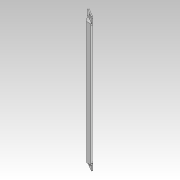
# Autodesk Inventor part: LedBracket
Saved by Autodesk Inventor 2020 (Build 240168000, 168)
## iProperties
Created: 2021-09-12
Part Number: LedBracket
Material: Generic
Document SubType Name: Modeling
Designer: DDeGo
Density: 1 g/cm^3
Appearance: Default
Author: DDeGo
Autodesk Inventor part; units mm, degrees
ref_plane "YZ Plane" through (0, 0, 0) normal (1, 0, 0) x (0, 1, 0)
ref_plane "XZ Plane" through (0, 0, 0) normal (0, 1, 0) x (-1, 0, 0)
ref_plane "XY Plane" through (0, 0, 0) normal (0, 0, 1) x (1, 0, 0)
sketch "Sketch1" plane through (0, 0, 0) normal (0, 0, 1) x (1, 0, 0)
  line L0 (-4, -105) -> (4, -105)
  line L1 (4, -105) -> (4, 105)
  line L2 (4, 105) -> (-4, 105)
  line L3 (-4, 105) -> (-4, -105)
  line L4 (-4, -105) -> (4, 105) construction
  line L5 (4, -105) -> (-4, 105) construction
  point P0 (0, 0)
  dimension "d0" = 8
  dimension "d1" = 210
  constraints: 12 end point, 2 midpoint, 2 parallel, 1 horizontal, 1 perpendicular
  measures "d0" distance of L1.end L2.end
  measures "d1" distance between parallel lines of L0 L2
extrude "Extrusion1" add sketch "Sketch1" along normal blind 2
sketch "Sketch2" plane through (-4, 105, 0) normal (0, 1, 0) x (1, 0, 0)
  line L0 (8, 0) -> (8, -2) projected
  line L1 (8, -2) -> (9.25, 0.1651)
  line L2 (9.25, 0.1651) -> (-8.0705, 10.1651)
  line L3 (8, -2) -> (0, -2) projected
  line L4 (0, 0) -> (0, -2) projected
  line L5 (8, -2) -> (0, -2)
  line L6 (0, -2) -> (-8.8205, 8.866)
  line L7 (-8.8205, 8.866) -> (-8.0705, 10.1651)
  point P0 (4, 0)
  dimension "d4" = 30
  dimension "d5" = 2.5
  dimension "d6" = 20
  dimension "d9" = 1.5
  constraints: 10 end point, 3 perpendicular
  measures "d4" angle of L2 L3
  measures "d5" distance from line of L0.end L2
  measures "d6" distance of L1.end L2.end
  measures "d9" distance of L6.end L2.end
extrude "Extrusion2" add sketch "Sketch2" along normal blind 2
sketch "Sketch3" plane through (-4, 107, 0) normal (0, 1, 0) x (1, 0, 0)
  line L0 (9.25, 0.1651) -> (-8.0705, 10.1651) projected
  line L1 (-8.8205, 8.866) -> (0, -2) projected
  line L2 (-8.0705, 10.1651) -> (-8.8205, 8.866)
  line L3 (-8.8205, 8.866) -> (8.5, -1.134)
  line L4 (8.5, -1.134) -> (9.25, 0.1651)
  line L5 (9.25, 0.1651) -> (-8.0705, 10.1651)
  line L6 (8, -2) -> (9.25, 0.1651) projected
  point P0 (4, 0)
  point P1 (9.25, 0.1651)
  constraints: 8 end point, 2 parallel, 1 perpendicular, 1 point on line
extrude "Extrusion3" add sketch "Sketch3" along normal blind 10
sketch "Sketch4" plane through (4.5, 107, 1.134) normal (-0.5, 0, 0.8660254) x (0.8660254, 0, 0.5)
  line L0 (-20, -2) -> (-20, 10) construction
  line L1 (-6.9282, 0) -> (0, 0) projected
  line L2 (-20, 10) -> (0, 0) construction
  circle A0 centre (-10, 5) radius 2.75
  point P0 (-4.4641, -107)
  dimension "d12" = 5.5
  constraints: 2 end point, 1 centre point, 1 midpoint
  measures "d12" diameter of A0
extrude "Extrusion4" cut sketch "Sketch4" against normal blind 10
fillet "Fillet1" radius 2 2 edges at (-12.4455, 117, -9.5155) (4.875, 117, 0.4845)
fillet "Fillet2" radius 5 1 edges at (0, 105, 0)
mirror "Mirror1" about plane through (0, 0, 0) normal (0, 1, 0) of "Extrusion2", "Extrusion3", "Extrusion4", "Fillet1", "Fillet2"
sketch "Sketch5" plane through (-4, 107, 0) normal (0, 1, 0) x (1, 0, 0)
  line L0 (0, -2) -> (8, -2) projected
  line L1 (4, -2) -> (350.4102, -202)
  line L2 (350.4102, -202) -> (-342.4102, -202)
  line L3 (-342.4102, -202) -> (4, -2)
  point P0 (4, 0)
  dimension "d17" = 120
  dimension "d18" = 200
  constraints: 6 end point, 1 equal length, 1 midpoint, 1 parallel
  measures "d17" angle of L3 L1
  measures "d18" distance between parallel lines of L0 L2
extrude "LED FOV" [suppressed]
body "Solid1"
